Autodesk Fusion 360 part; units mm, degrees
note: some values were not read from the file. Chosen so that the rebuilt part matches the saved one: which face or edge a step refers to; that a step has no effect; which bodies a step acts on; which pieces of a blend or face edit are solid.
(part 2 of 2)
sketch "Sketch80" plane through (0, 0, 95) normal (0, 0, 1) x (-1, 0, 0)
  line L0 (-110, -10) -> (-100, -10)
  line L1 (-100, -10) -> (-100, 20)
  line L2 (-100, 20) -> (-110, 20)
  line L3 (-110, 20) -> (-110, -10)
  line L4 (-110, 20) -> (-100, 20)
  line L5 (-100, 20) -> (-100, 10)
  line L6 (-100, 10) -> (-110, 10)
  line L7 (-110, 10) -> (-110, 20)
  line L8 (-110, 0) -> (-100, 0)
  line L9 (-100, 0) -> (-100, -10)
  line L10 (-100, -10) -> (-110, -10)
  line L11 (-110, -10) -> (-110, 0)
  constraint horizontal L4
  constraint vertical L5
  constraint horizontal L6
  constraint vertical L7
  constraint coincident L1 L5.end
  constraint coincident L2.end L3.start
  constraint horizontal L8
  constraint vertical L9
  constraint horizontal L10
  constraint vertical L11
  constraint coincident L3 L8.start
extrude "Extrude63" add sketch "Sketch80" along normal blind 40 contours L0 L1 L3 L8 L9 L10 L11 | L1 L2 L3 L4 L5 L6 L7 bodies 1
sketch "Sketch81" plane through (0, 0, 0) normal (0, -1, 0) x (1, 0, 0)
  line L0 (100, 95) -> (110, 95)
  line L1 (110, 95) -> (110, 135)
  line L2 (110, 135) -> (100, 135)
  line L3 (100, 135) -> (100, 95)
  line L4 (100, 135) -> (110, 135)
  line L5 (110, 135) -> (110, 125)
  line L6 (110, 125) -> (100, 125)
  line L7 (100, 125) -> (100, 135)
  constraint horizontal L4
  constraint vertical L5
  constraint horizontal L6
  constraint vertical L7
  constraint coincident L1 L5.end
  constraint coincident L2.end L3.start
extrude "Extrude64" add sketch "Sketch81" along normal blind 10 contours L1 L2 L3 L4 L5 L6 L7 bodies 1
sketch "Sketch82" plane through (0, 0, 85) normal (0, 0, 1) x (1, 0, 0)
  line L0 (110, 20) -> (100, 20)
  line L1 (100, 20) -> (100, 40)
  line L2 (100, 40) -> (110, 40)
  line L3 (110, 40) -> (110, 20)
  constraint horizontal L0
  constraint vertical L1
  constraint horizontal L2
  constraint vertical L3
extrude "Extrude65" add sketch "Sketch82" along normal blind 10 bodies 1
sketch "Sketch83" plane through (0, 0, 95) normal (0, 0, 1) x (-1, 0, 0)
  line L0 (-110, -40) -> (-100, -40)
  line L1 (-100, -40) -> (-100, -20)
  line L2 (-100, -20) -> (-110, -20)
  line L3 (-110, -20) -> (-110, -40)
  line L4 (-100, -40) -> (-110, -40)
  line L5 (-110, -40) -> (-110, -30)
  line L6 (-110, -30) -> (-100, -30)
  line L7 (-100, -30) -> (-100, -40)
  constraint horizontal L4
  constraint vertical L5
  constraint horizontal L6
  constraint vertical L7
  constraint midpoint L3 L5.end
  constraint coincident L0.end L1.start
extrude "Extrude66" add sketch "Sketch83" along normal blind 40 contours L0 L1 L3 L4 L5 L6 L7 bodies 1
sketch "Sketch84" plane through (0, 30, 0) normal (0, -1, 0) x (1, 0, 0)
  line L0 (100, 95) -> (110, 95)
  line L1 (110, 95) -> (110, 135)
  line L2 (110, 135) -> (100, 135)
  line L3 (100, 135) -> (100, 95)
  line L4 (100, 135) -> (110, 135)
  line L5 (110, 135) -> (110, 125)
  line L6 (110, 125) -> (100, 125)
  line L7 (100, 125) -> (100, 135)
  line L8 (100, 120) -> (110, 120)
  line L9 (110, 120) -> (110, 110)
  line L10 (110, 110) -> (100, 110)
  line L11 (100, 110) -> (100, 120)
  dimension "d267" = 10
  dimension "d268" = 10
  constraint horizontal L4
  constraint vertical L5
  constraint horizontal L6
  constraint vertical L7
  constraint coincident L2.end L3.start
  constraint horizontal L8
  constraint vertical L9
  constraint horizontal L10
  constraint vertical L11
  constraint coincident L1 L9.end
  constraint coincident L3 L8.start
  measures "d267" distance of L2.end L1.end
  measures "d268" distance of L2.end L6.end
extrude "Extrude67" add sketch "Sketch84" along normal blind 10 contours L1 L3 L8 L9 L10 L11 | L1 L2 L3 L4 L5 L6 L7 bodies 1
sketch "Sketch85" plane through (0, 0, 85) normal (0, 0, 1) x (1, 0, 0)
sketch "Sketch86" plane through (0, 0, 85) normal (0, 0, 1) x (1, 0, 0)
  line L0 (110, 50) -> (100, 50)
  line L1 (100, 50) -> (100, 60)
  line L2 (100, 60) -> (110, 60)
  line L3 (110, 60) -> (110, 50)
  constraint horizontal L0
  constraint vertical L1
  constraint horizontal L2
  constraint vertical L3
extrude "Extrude68" add sketch "Sketch86" along normal blind 50 bodies 1
sketch "Sketch87" plane through (0, 0, 85) normal (0, 0, 1) x (-1, 0, 0)
sketch "Sketch88" plane through (0, 0, 85) normal (0, 0, 1) x (1, 0, 0)
sketch "Sketch89" plane through (0, 0, 85) normal (0, 0, 1) x (-1, 0, 0)
  line L0 (-110, -65) -> (-100, -65)
  line L1 (-100, -65) -> (-100, -85)
  line L2 (-100, -85) -> (-110, -85)
  line L3 (-110, -85) -> (-110, -65)
  constraint horizontal L0
  constraint vertical L1
  constraint horizontal L2
  constraint vertical L3
extrude "Extrude69" add sketch "Sketch89" along normal blind 10 bodies 1
sketch "Sketch90" plane through (0, 0, 95) normal (0, 0, 1) x (-1, 0, 0)
  line L0 (-110, -85) -> (-100, -85)
  line L1 (-100, -85) -> (-100, -65)
  line L2 (-100, -65) -> (-110, -65)
  line L3 (-110, -65) -> (-110, -85)
  line L4 (-100, -85) -> (-110, -85)
  line L5 (-110, -85) -> (-110, -75)
  line L6 (-110, -75) -> (-100, -75)
  line L7 (-100, -75) -> (-100, -85)
  constraint horizontal L4
  constraint vertical L5
  constraint horizontal L6
  constraint vertical L7
  constraint coincident L0.end L1.start
extrude "Extrude70" add sketch "Sketch90" along normal blind 40 contours L0 L1 L3 L4 L5 L6 L7 bodies 1
sketch "Sketch91" plane through (0, 75, 0) normal (0, -1, 0) x (1, 0, 0)
  line L0 (100, 95) -> (110, 95)
  line L1 (110, 95) -> (110, 135)
  line L2 (110, 135) -> (100, 135)
  line L3 (100, 135) -> (100, 95)
  line L4 (100, 135) -> (110, 135)
  line L5 (110, 135) -> (110, 125)
  line L6 (110, 125) -> (100, 125)
  line L7 (100, 125) -> (100, 135)
  line L8 (100, 119) -> (110, 119)
  line L9 (110, 119) -> (110, 109)
  line L10 (110, 109) -> (100, 109)
  line L11 (100, 109) -> (100, 119)
  dimension "d277" = 10
  dimension "d278" = 10
  constraint horizontal L4
  constraint vertical L5
  constraint horizontal L6
  constraint vertical L7
  constraint coincident L2.end L3.start
  constraint horizontal L8
  constraint vertical L9
  constraint horizontal L10
  constraint vertical L11
  constraint coincident L3 L8.start
  measures "d277" distance of L8.start L8.end
  measures "d278" distance of L8.start L10.end
extrude "Extrude71" add sketch "Sketch91" along normal blind 10 contours L1 L3 L8 L9 L10 L11 | L1 L2 L3 L4 L5 L6 L7 bodies 1
sketch "Sketch92" plane through (0, 0, 85) normal (0, 0, 1) x (1, 0, 0)
  line L0 (-140, 90) -> (-120, 90)
  line L1 (-120, 90) -> (-120, -80)
  line L2 (-120, -80) -> (-140, -80)
  line L3 (-140, -80) -> (-140, 90)
  constraint horizontal L0
  constraint vertical L1
  constraint horizontal L2
  constraint vertical L3
extrude "Extrude72" add sketch "Sketch92" along normal blind 10 bodies 1
sketch "Sketch93" plane through (0, 0, 95) normal (0, 0, 1) x (-1, 0, 0)
  line L0 (140, 80) -> (120, 80)
  line L1 (120, 80) -> (120, -90)
  line L2 (120, -90) -> (140, -90)
  line L3 (140, -90) -> (140, 80)
  line L4 (140, -60) -> (120, -60)
  line L5 (120, -60) -> (120, -40)
  line L6 (120, -40) -> (140, -40)
  line L7 (140, -40) -> (140, -60)
  line L8 (120, 50) -> (140, 50)
  line L9 (140, 50) -> (140, 30)
  line L10 (140, 30) -> (120, 30)
  line L11 (120, 30) -> (120, 50)
  constraint horizontal L4
  constraint vertical L5
  constraint horizontal L6
  constraint vertical L7
  constraint coincident L3 L4.start
  constraint horizontal L8
  constraint vertical L9
  constraint horizontal L10
  constraint vertical L11
  constraint coincident L1 L8.start
extrude "Extrude73" add sketch "Sketch93" along normal blind 50 contours L1 L3 L8 L9 L10 L11 | L1 L3 L4 L5 L6 L7 bodies 1
sketch "Sketch94" plane through (0, 0, 145) normal (0, 0, 1) x (-1, 0, 0)
  line L0 (140, -40) -> (120, -40)
  line L1 (120, -40) -> (120, -60)
  line L2 (120, -60) -> (140, -60)
  line L3 (140, -60) -> (140, -40)
  line L4 (140, -110) -> (120, -110)
  line L5 (120, -110) -> (120, 100)
  line L6 (120, 100) -> (140, 100)
  line L7 (140, 100) -> (140, -110)
  constraint horizontal L4
  constraint vertical L5
  constraint horizontal L6
  constraint vertical L7
extrude "Extrude74" add sketch "Sketch94" along normal blind 10 bodies 1
sketch "Sketch95" plane through (0, -100, 0) normal (0, -1, 0) x (1, 0, 0)
  line L0 (-140, 145) -> (-120, 145)
  line L1 (-120, 145) -> (-120, 155)
  line L2 (-120, 155) -> (-140, 155)
  line L3 (-140, 155) -> (-140, 145)
  line L4 (-115, 160) -> (-145, 160)
  line L5 (-145, 160) -> (-145, 140)
  line L6 (-145, 140) -> (-115, 140)
  line L7 (-115, 140) -> (-115, 160)
  line L8 (-115, 160) -> (-145, 140) construction
  line L9 (-145, 160) -> (-115, 140) construction
  point P0 (-130, 150)
  dimension "d307" = 30
  dimension "d308" = 20
  constraint horizontal L4
  constraint perpendicular L4 L5
  constraint parallel L4 L6
  constraint parallel L5 L7
  constraint coincident L8 P0
  constraint coincident L9 P0
  measures "d307" distance of L5.end L6.end
  measures "d308" distance of L4.end L5.end
extrude "Extrude75" add sketch "Sketch95" along normal blind 10 contours L0 L1 L2 L3 | L4 L5 L6 L7 bodies 1
sketch "Sketch96" plane through (0, 110, 0) normal (0, 1, 0) x (-1, 0, 0)
  line L0 (120, 145) -> (140, 145)
  line L1 (140, 145) -> (140, 155)
  line L2 (140, 155) -> (120, 155)
  line L3 (120, 155) -> (120, 145)
  line L4 (145, 140) -> (115, 140)
  line L5 (115, 140) -> (115, 160)
  line L6 (115, 160) -> (145, 160)
  line L7 (145, 160) -> (145, 140)
  line L8 (145, 140) -> (115, 160) construction
  line L9 (115, 140) -> (145, 160) construction
  point P0 (130, 150)
  dimension "d311" = 30
  dimension "d312" = 20
  constraint horizontal L4
  constraint perpendicular L4 L5
  constraint parallel L4 L6
  constraint parallel L5 L7
  constraint coincident L8 P0
  constraint coincident L9 P0
  measures "d311" distance of L5.end L6.end
  measures "d312" distance of L4.end L5.end
extrude "Extrude76" add sketch "Sketch96" along normal blind 10 contours L0 L1 L2 L3 | L4 L5 L6 L7 bodies 1
copy_body "Body->Comp25" bodies 1 removing the originals makes body 14 in component "base_link"
component "right_wheel1" placed x (0, 0, 1) y (0, 1, 0) z (-1, 0, 0) at (200, 0, -20)
component "right_wheel2" placed x (1, 0, 0) y (0, 1, 0) z (0, 0, 1) at (-75, 0, 5)
component "left_wheel1" placed x (1, 0, 0) y (0, 1, 0) z (0, 0, 1) at (75, 0, 5)
component "left_wheel2" placed x (1, 0, 0) y (0, 1, 0) z (0, 0, 1) at (-75, 0, 5)
component "lidar" placed x (1, 0, 0) y (0, 1, 0) z (0, 0, 1) at (0, 0, 0)
component "base_link" placed x (1, 0, 0) y (0, 1, 0) z (0, 0, 1) at (0, 0, 0)
named bodies: "base_link", "right_wheel1", "right_wheel2", "left_wheel1", "left_wheel2", "lidar"
